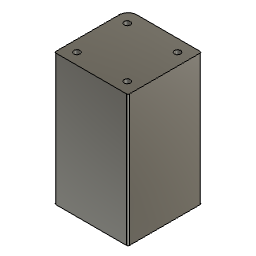
Leg_Extension_Rear_x2 (Autodesk Fusion 360 design; units mm, degrees)
Autodesk Fusion 360 part; units mm, degrees
note: some values were not read from the file. Set by a fixed rule: which sketch regions a step uses.
sketch "Skizze1" plane through (0, 0, 0) normal (0, 0, 1) x (1, 0, 0)
  line L0 (0, 0) -> (50.5, 0)
  line L1 (50.5, 0) -> (50.5, 50.5)
  line L2 (50.5, 50.5) -> (0, 50.5)
  line L3 (0, 50.5) -> (0, 0)
  line L4 (50.5, 0) -> (50.5, 5)
  line L5 (50.5, 5) -> (50.5, 8.5)
  line L6 (50.5, 8.5) -> (50.5, 13.5)
  circle A0 centre (25, 25) radius 12.7
  line L7 (42.25, 42.25) -> (7.75, 42.25)
  line L8 (7.75, 42.25) -> (7.75, 7.75)
  line L9 (7.75, 7.75) -> (42.25, 7.75)
  line L10 (42.25, 7.75) -> (42.25, 42.25)
  line L11 (42.25, 42.25) -> (7.75, 7.75) construction
  line L12 (7.75, 42.25) -> (42.25, 7.75) construction
  point P0 (25, 25)
  dimension "d1" = 50.5
  dimension "d2" = 50.5
  dimension "d17" = 25.4
  dimension "d18" = 34.5
  dimension "d19" = 34.5
  constraint horizontal L0
  constraint horizontal L2
  constraint vertical L3
  constraint coincident L0.start L3.end
  constraint perpendicular L7 L8
  constraint parallel L7 L9
  constraint parallel L8 L10
  constraint horizontal L7
  constraint coincident L11 P0
  constraint coincident L12 P0
  constraint coincident P0 A0.centre
  measures "d1" distance of L0.start L0.end
  measures "d2" distance of L0.start L2.end
  measures "d17" diameter of A0
  measures "d18" distance of L8.end L9.end
  measures "d19" distance of L7.end L8.end
extrude "Extrusion1" add sketch "Skizze1" along normal blind 90 contours L0 L1 L2 L3 L4 L5 L6 | A0 | L7 L8 L9 L10
extrude "Extrusion2" cut sketch "Skizze1" along normal blind 15 contours A0
chamfer "Fase1" distance 2.5 distance2 15 1 edges at (13.1594, 20.4075, 0) measured on face at (25.483, 46.2215, 0)
sketch "Skizze2" plane through (0, 0, 0) normal (0, 0, -1) x (1, 0, 0)
  line L0 (0, 0) -> (0, -50.5)
  line L1 (0, -50.5) -> (50.5, -50.5)
  line L2 (50.5, -50.5) -> (50.5, 0)
  line L3 (50.5, 0) -> (0, 0)
  circle A0 centre (25, -25) radius 15.2
  line L4 (42.25, -7.75) -> (7.75, -7.75)
  line L5 (7.75, -7.75) -> (7.75, -42.25)
  line L6 (7.75, -42.25) -> (42.25, -42.25)
  line L7 (42.25, -42.25) -> (42.25, -7.75)
  line L8 (42.25, -7.75) -> (7.75, -42.25) construction
  line L9 (7.75, -7.75) -> (42.25, -42.25) construction
  point P0 (25, -25)
  dimension "d26" = 34.5
  dimension "d27" = 34.5
  constraint perpendicular L4 L5
  constraint parallel L4 L6
  constraint parallel L5 L7
  constraint horizontal L4
  constraint coincident L8 P0
  constraint coincident L9 P0
  constraint coincident P0 A0.centre
  measures "d26" distance of L5.end L6.end
  measures "d27" distance of L4.end L5.end
hole "Bohrung1" at (7.75, 7.75, 0) at (7.75, 42.25, 0) at (42.25, 42.25, 0) at (42.25, 7.75, 0) direction (0, 0, 1) diameter 8.8 depth 82 tip angle 180
hole "Bohrung2" at (7.75, 42.25, 82) direction (0, 0, 1) diameter 4.2 depth 82 tip angle 180 countersink diameter 8.6 countersink angle 90
hole "Bohrung3" at (7.75, 7.75, 82) direction (0, 0, 1) diameter 4.2 depth 82 tip angle 180 countersink diameter 8.6 countersink angle 90
hole "Bohrung4" at (42.25, 7.75, 82) direction (0, 0, 1) diameter 4.2 depth 82 tip angle 180 countersink diameter 8.6 countersink angle 90
hole "Bohrung5" at (42.25, 42.25, 82) direction (0, 0, 1) diameter 4.2 depth 82 tip angle 180 countersink diameter 8.6 countersink angle 90
fillet "Fillet3" radius 6 1 edges at (0, 50.5, 45)
fillet "Fillet4" radius 1 3 edges at (0, 0, 45) (50.5, 0, 45) (50.5, 50.5, 45)
